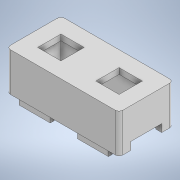
# Autodesk Inventor part: Keyboard_Base
Saved by Autodesk Inventor 2021 (Build 250183000, 183)
## iProperties
Created: 2020-07-07
Part Number: Keyboard_Base
Material: Generic
Document SubType Name: Modeling
Designer: ameli
Density: 1 g/cm^3
Appearance: Default
Author: ameli
Autodesk Inventor part; units mm, degrees
ref_plane "YZ Plane" through (0, 0, 0) normal (1, 0, 0) x (0, 1, 0)
ref_plane "XZ Plane" through (0, 0, 0) normal (0, 1, 0) x (-1, 0, 0)
ref_plane "XY Plane" through (0, 0, 0) normal (0, 0, 1) x (1, 0, 0)
sketch "Sketch1" plane through (0, 0, 0) normal (0, 1, 0) x (-1, 0, 0)
  line L0 (14.5, 7) -> (-14.5, 7)
  line L1 (-14.5, 7) -> (-14.5, -7)
  line L2 (-14.5, -7) -> (14.5, -7)
  line L3 (14.5, -7) -> (14.5, 7)
  point P0 (0, 0)
  dimension "d0" = 14
  dimension "d1" = 29
  dimension "d2" = 14.5
  dimension "d3" = 7
  constraints: 8 end point, 2 parallel, 1 horizontal, 1 perpendicular
  measures "d0" distance of L2.end L0.start
  measures "d1" distance of L1.end L2.end
  measures "d2" distance from line of point (0, 0) L3
  measures "d3" distance from line of point (0, 0) L2
extrude "Extrusion1" add sketch "Sketch1" along normal blind 10
fillet "Fillet1" radius 1 4 edges at (14.5, 5, 7) (14.5, 5, -7) (-14.5, 5, -7) (-14.5, 5, 7)
shell "Shell1" thickness 1.5 removed faces 1 at (4.5, 0, 2.3333)
sketch "Sketch3" plane through (0, 10, 0) normal (0, 1, 0) x (1, 0, 0)
  line L0 (-10.5, -3) -> (-4.5, -3)
  line L1 (-4.5, -3) -> (-4.5, 3)
  line L2 (-4.5, 3) -> (-10.5, 3)
  line L3 (-10.5, 3) -> (-10.5, -3)
  line L4 (4.5, -3) -> (10.5, -3)
  line L5 (10.5, -3) -> (10.5, 3)
  line L6 (10.5, 3) -> (4.5, 3)
  line L7 (4.5, 3) -> (4.5, -3)
  line L8 (-13.5, -7) -> (13.5, -7) projected
  line L9 (-14.5, 6) -> (-14.5, -6) projected
  line L10 (14.5, -6) -> (14.5, 6) projected
  point P0 (0, 0)
  dimension "d14" = 6
  dimension "d15" = 6
  dimension "d16" = 4
  dimension "d17" = 4
  dimension "d18" = 4
  dimension "d19" = 6
  constraints: 16 end point, 4 parallel, 2 horizontal, 2 perpendicular, 2 point on line
  measures "d14" distance of L2.end L0.start
  measures "d15" distance of L1.end L2.end
  measures "d16" distance between parallel lines of L8 L0
  measures "d17" distance between parallel lines of L9 L3
  measures "d18" distance between parallel lines of L10 L5
  measures "d19" distance of L5.end L6.end
extrude "Extrusion3" cut sketch "Sketch3" against normal through all
sketch "Sketch4" plane through (0, 0, 0) normal (0, -1, 0) x (1, 0, 0)
  line L0 (11.5, 6.75) -> (3.5, 6.75)
  line L1 (3.5, 6.75) -> (3.5, 5.75)
  line L2 (3.5, 5.75) -> (11.5, 5.75)
  line L3 (11.5, 5.75) -> (11.5, 6.75)
  line L4 (-3.5, 6.75) -> (-11.5, 6.75)
  line L5 (-11.5, 6.75) -> (-11.5, 5.75)
  line L6 (-11.5, 5.75) -> (-3.5, 5.75)
  line L7 (-3.5, 5.75) -> (-3.5, 6.75)
  line L8 (11.5, -5.75) -> (3.5, -5.75)
  line L9 (3.5, -5.75) -> (3.5, -6.75)
  line L10 (3.5, -6.75) -> (11.5, -6.75)
  line L11 (11.5, -6.75) -> (11.5, -5.75)
  line L12 (-3.5, -5.75) -> (-11.5, -5.75)
  line L13 (-11.5, -5.75) -> (-11.5, -6.75)
  line L14 (-11.5, -6.75) -> (-3.5, -6.75)
  line L15 (-3.5, -6.75) -> (-3.5, -5.75)
  line L16 (14.5, 6) -> (14.5, -6) projected
  line L17 (-14.5, -6) -> (-14.5, 6) projected
  line L18 (-13, 5.5) -> (13, 5.5) projected
  line L19 (13.5, -7) -> (-13.5, -7) projected
  point P0 (0, 0)
  dimension "d22" = 3
  dimension "d23" = 3
  dimension "d24" = 1
  dimension "d25" = 8
  dimension "d26" = 1
  dimension "d27" = 8
  dimension "d28" = 0.25
  dimension "d29" = 0.25
  constraints: 32 end point, 8 parallel, 8 point on line, 4 horizontal, 4 perpendicular
  measures "d22" distance between parallel lines of L16 L3
  measures "d23" distance between parallel lines of L17 L5
  measures "d24" distance of L6.end L4.start
  measures "d25" distance of L5.end L6.end
  measures "d26" distance of L14.end L12.start
  measures "d27" distance of L9.end L10.end
  measures "d28" distance between parallel lines of L18 L2
  measures "d29" distance between parallel lines of L19 L10
extrude "Extrusion4" add sketch "Sketch4" along normal blind 1.5
sketch "Sketch5" plane through (14.5, 0, 6) normal (1, 0, 0) x (0, 0, -1)
  line L0 (0, 0) -> (12, 0) projected
  line L1 (2, 2) -> (10, 2)
  line L2 (10, 2) -> (10, 0)
  line L3 (10, 0) -> (2, 0)
  line L4 (2, 0) -> (2, 2)
  line L5 (0, 0) -> (0, 10) projected
  point P0 (6, 0)
  point P1 (2, 0)
  dimension "d32" = 8
  dimension "d33" = 2
  dimension "d34" = 2
  constraints: 8 end point, 2 parallel, 1 horizontal, 1 perpendicular, 1 point on line
  measures "d32" distance of L1.start L1.end
  measures "d33" distance of L3.end L1.start
  measures "d34" distance between parallel lines of L5 L4
extrude "Extrusion5" cut sketch "Sketch5" against normal blind 1.5
body "Solid1"
